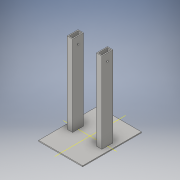
# Autodesk Inventor part: PostForLift
Saved by Autodesk Inventor 2016 SP1 (Build 200210100, 210)
## iProperties
Created: 2016-02-01
Part Number: PostForLift
Material: Generic
Document SubType Name: Modeling
Designer: steele
Density: 1 g/cm^3
Appearance: Default
Author: steele
Autodesk Inventor part; units mm, degrees
ref_plane "YZ Plane" through (0, 0, 0) normal (1, 0, 0) x (0, 1, 0)
ref_plane "XZ Plane" through (0, 0, 0) normal (0, 1, 0) x (-1, 0, 0)
ref_plane "XY Plane" through (0, 0, 0) normal (0, 0, 1) x (1, 0, 0)
sketch "Sketch1" plane through (0, 0, 0) normal (0, 1, 0) x (-1, 0, 0)
  line L0 (76.2, 101.6) -> (-76.2, 101.6)
  line L1 (-76.2, 101.6) -> (-76.2, -101.6)
  line L2 (-76.2, -101.6) -> (76.2, -101.6)
  line L3 (76.2, -101.6) -> (76.2, 101.6)
  line L4 (76.2, 101.6) -> (-76.2, -101.6) construction
  line L5 (-76.2, 101.6) -> (76.2, -101.6) construction
  point P0 (0, 0)
  dimension "d0" = 152.4
  dimension "d1" = 203.2
  constraints: 12 end point, 2 midpoint, 2 parallel, 1 horizontal, 1 perpendicular
  measures "d0" distance of L0.start L0.end
  measures "d1" distance of L2.end L0.start
extrude "Extrusion1" add sketch "Sketch1" against normal blind 3.175
sketch "Sketch2" plane through (0, 0, 0) normal (0, 1, 0) x (1, 0, 0)
  line L0 (-60.325, -19.05) -> (-41.275, -19.05)
  line L1 (-41.275, -19.05) -> (-41.275, 19.05)
  line L2 (-41.275, 19.05) -> (-60.325, 19.05)
  line L3 (-60.325, 19.05) -> (-60.325, -19.05)
  line L4 (-60.325, -19.05) -> (-41.275, 19.05) construction
  line L5 (-41.275, -19.05) -> (-60.325, 19.05) construction
  line L6 (-57.15, -15.875) -> (-44.45, -15.875)
  line L7 (-44.45, -15.875) -> (-44.45, 15.875)
  line L8 (-44.45, 15.875) -> (-57.15, 15.875)
  line L9 (-57.15, 15.875) -> (-57.15, -15.875)
  line L10 (-57.15, -15.875) -> (-44.45, 15.875) construction
  line L11 (-44.45, -15.875) -> (-57.15, 15.875) construction
  line L12 (-76.2, 101.6) -> (76.2, 101.6) construction
  line L13 (0, 101.6) -> (0, -101.6) construction
  line L14 (60.325, -19.05) -> (41.275, -19.05)
  line L15 (41.275, -19.05) -> (41.275, 19.05)
  line L16 (41.275, 19.05) -> (60.325, 19.05)
  line L17 (60.325, 19.05) -> (60.325, -19.05)
  line L18 (57.15, -15.875) -> (44.45, -15.875)
  line L19 (44.45, -15.875) -> (44.45, 15.875)
  line L20 (44.45, 15.875) -> (57.15, 15.875)
  line L21 (57.15, 15.875) -> (57.15, -15.875)
  point P0 (0, 0)
  point P1 (-50.8, 0)
  dimension "d4" = 50.8
  dimension "d5" = 19.05
  dimension "d6" = 38.1
  dimension "d7" = 3.175
  dimension "d8" = 3.175
  constraints: 42 end point, 8 symmetric about line, 5 midpoint, 4 parallel, 2 horizontal, 2 perpendicular, 1 vertical
  measures "d4" distance of point (0, 0) point (-50.8, 0)
  measures "d5" distance of L0.start L0.end
  measures "d6" distance of L2.end L0.start
  measures "d7" distance between parallel lines of L0 L6
  measures "d8" distance between parallel lines of L9 L3
extrude "Extrusion2" add sketch "Sketch2" along normal blind 279.4
sketch "Sketch3" plane through (-60.325, 0, -19.05) normal (-1, 0, 0) x (0, 0, 1)
  line L0 (0, 279.4) -> (38.1, 279.4) construction
  line L1 (19.05, 279.4) -> (19.05, 0) construction
  circle A0 centre (19.05, 254) radius 3.175
  line L2 (-82.55, 0) -> (120.65, 0) projected
  dimension "d11" = 6.35
  dimension "d12" = 254
  constraints: 2 end point, 1 centre point, 1 midpoint, 1 point on line, 1 vertical
  measures "d11" diameter of A0
  measures "d12" distance from line of A0.centre L2
extrude "Extrusion3" cut sketch "Sketch3" against normal through all
equation "\"d0\" = BaseWidth"
equation "\"d1\" = BaseLength"
equation "\"d2\" = BaseThickness"
equation "\"d4\" = postCenterDistanceFromCenterOfBase"
equation "\"d5\" = postWidth"
equation "\"d6\" = postLength"
equation "\"d7\" = postThickness"
equation "\"d8\" = postThickness"
equation "\"d9\" = postHeight"
equation "\"d11\" = axelDiam"
equation "\"d12\" = axelHeightAbovePlate"
equation "\"BaseWidth\" = 152.4"
equation "\"BaseLength\" = 203.2"
equation "\"BaseThickness\" = 3.175"
equation "\"postWidth\" = 19.05"
equation "\"postLength\" = 38.1"
equation "\"postThickness\" = 3.175"
equation "\"postCenterDistanceFromCenterOfBase\" = 50.8"
equation "\"axelDiam\" = 6.35"
equation "\"axelHeightAbovePlate\" = 254"
equation "\"postHeight\" = 279.4"
body "Solid1"
